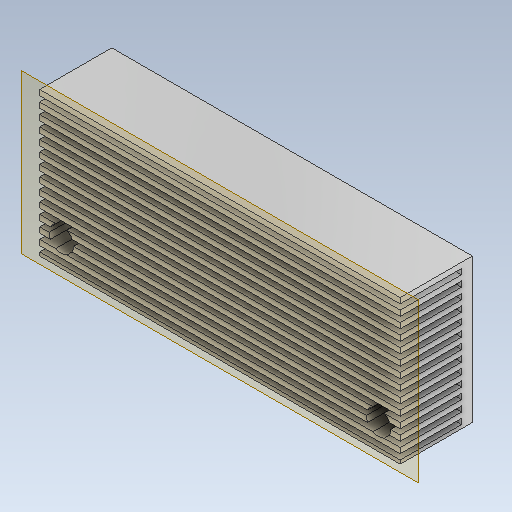
# Autodesk Inventor part: ExternalHeatSinkandClamp
Saved by Autodesk Inventor 2021 (Build 250183000, 183)
## iProperties
Created: 2021-10-17
Part Number: ExternalHeatSinkandClamp
Material: Generic
Document SubType Name: Sheet Metal
Designer: Unit-005
Density: 1 g/cm^3
Sheet Metal Rule: Default
Appearance: Default
Author: Unit-005
Autodesk Inventor part; units mm, degrees
ref_plane "YZ Plane" through (0, 0, 0) normal (1, 0, 0) x (0, 1, 0)
ref_plane "XZ Plane" through (0, 0, 0) normal (0, 1, 0) x (-1, 0, 0)
sketch "Sketch1" plane through (0, 0, 0) normal (0, 0, 1) x (1, 0, 0)
  line L0 (-50, 20) -> (50, 20)
  line L1 (50, 20) -> (50, -20)
  line L2 (50, -20) -> (-50, -20)
  line L3 (-50, -20) -> (-50, 20)
  line L4 (-50, 20) -> (50, -20) construction
  line L5 (50, 20) -> (-50, -20) construction
  point P0 (0, 0)
  dimension "d0" = 100
  dimension "d1" = 40
  constraints: 12 end point, 2 midpoint, 2 parallel, 1 horizontal, 1 perpendicular
  measures "d0" distance of L1.end L2.end
  measures "d1" distance of L0.end L1.end
extrude "Extrusion1" add sketch "Sketch1" along normal blind 20
sketch "Sketch2" plane through (0, 0, 20) normal (0, 0, 1) x (1, 0, 0)
  line L0 (-50, -20) -> (50, -20) projected
  line L1 (50, -20) -> (50, 20) projected
  line L2 (50, 20) -> (-50, 20) projected
  line L3 (-50, 20) -> (-50, -20) projected
  line L4 (-70, 0) -> (70, 0) projected
  line L5 (0, -28) -> (0, 28) projected
  line L6 (50, -20) -> (50, 20) projected
  line L7 (-50, 17) -> (50, 17)
  line L8 (50, 17) -> (50, 18.5)
  line L9 (50, 18.5) -> (-50, 18.5)
  line L10 (-50, 18.5) -> (-50, 17)
  line L11 (-50, 17) -> (50, 18.5) construction
  line L12 (50, 17) -> (-50, 18.5) construction
  point P0 (0, 0)
  point P1 (0, 17.75)
  dimension "d4" = 1.5
  dimension "d6" = 1.5
  constraints: 12 end point, 2 midpoint, 2 parallel, 2 point on line, 1 horizontal, 1 perpendicular
  measures "d4" distance of L8.end L7.end
  measures "d6" distance between parallel lines of L2 L9
extrude "Extrusion2" cut sketch "Sketch2" against normal blind 17 contours L3 L9 L5 L7 | L5 L9 L1 L7
pattern_linear "Rectangular Pattern1" count 13 spacing 3 along (0, -1, 0) of "Extrusion2"
ref_plane "Work Plane1" through (0, 0, 20) normal (0, 0, 1) x (1, 0, 0)
sketch "Sketch4" plane through (0, 0, 20) normal (0, 0, 1) x (1, 0, 0)
  line L0 (0, -28) -> (0, 28) projected
  line L1 (50, 0.5) -> (50, -1) projected
  line L2 (50, 20) -> (-50, 20) projected
  line L3 (-50, -20) -> (50, -20) projected
  line L4 (-50, -4) -> (-50, -5.5) projected
  point P0 (0, 0)
  point P1 (44, -13)
  point P2 (-44, -13)
  dimension "d22" = 6
  dimension "d30" = 7
  dimension "d31" = 7
  dimension "d32" = 6
  measures "d22" distance from line of L1 point (44, -13)
  measures "d30" distance from line of L3 point (44, -13)
  measures "d31" distance from line of L3 point (-44, -13)
  measures "d32" distance from line of L4 point (-44, -13)
hole "Hole2" at (44, -13, 20) at (-44, -13, 20) direction (0, 0, -1) diameter 6.756 end through all clearance for "Socket Head Cap Screw" size "1/4" standard "Ansi Unified Screw Threads"
equation "\"d28\" = Thickness"
equation "\"BendRadius\" = Thickness"
equation "\"BendReliefWidth\" = Thickness"
equation "\"BendReliefDepth\" = 0.5 * Thickness"
equation "\"CornerReliefSize\" = 4 * Thickness"
equation "\"MinimumRemnant\" = 2 * Thickness"
equation "\"TransitionRadius\" = BendRadius"
equation "\"JacobiRadiusSize\" = BendRadius"
equation "\"GapSize\" = Thickness"
equation "\"Thickness\" = 3.048"
body "Solid1"
